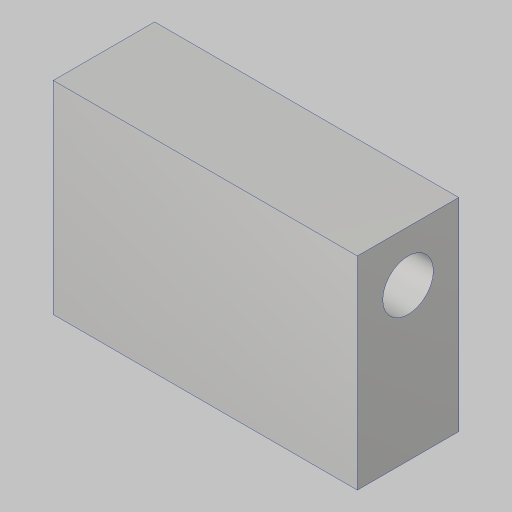
# Autodesk Inventor part: CHD-001
Saved by Autodesk Inventor 2023.5 (Build 275446000, 446)
## iProperties
Created: 2025-01-30
Part Number: CHD-001
Material: Aluminum 6061
Document SubType Name: Modeling
Designer: slick
Density: 2.7 g/cm^3
Appearance: Aluminum - Flat
Author: slick
Autodesk Inventor part; units mm, degrees
ref_plane "YZ Plane" through (0, 0, 0) normal (1, 0, 0) x (0, 1, 0)
ref_plane "XZ Plane" through (0, 0, 0) normal (0, 1, 0) x (-1, 0, 0)
ref_plane "XY Plane" through (0, 0, 0) normal (0, 0, 1) x (1, 0, 0)
sketch "Sketch1" plane through (0, 0, 0) normal (1, 0, 0) x (0, 1, 0)
  line L0 (25.4, 12.7) -> (-25.4, 12.7)
  line L1 (-25.4, 12.7) -> (-25.4, -12.7)
  line L2 (-25.4, -12.7) -> (25.4, -12.7)
  line L3 (25.4, -12.7) -> (25.4, 12.7)
  line L4 (25.4, 12.7) -> (-25.4, -12.7) construction
  line L5 (-25.4, 12.7) -> (25.4, -12.7) construction
  point P0 (0, 0)
  dimension "d0" = 50.8
  dimension "d1" = 25.4
  constraints: 12 end point, 2 midpoint, 2 parallel, 1 horizontal, 1 perpendicular
  measures "d0" distance of L2.end L1.end
  measures "d1" distance of L1.end L0.end
extrude "Extrusion1" add sketch "Sketch1" along normal blind 76.2
sketch "Sketch2" plane through (76.2, 0, 0) normal (1, 0, 0) x (0, 0, -1)
  line L0 (12.7, 25.4) -> (-12.7, 25.4) construction
  point P0 (0, 0)
  point P1 (0, 12.7)
  dimension "d4" = 12.7
  constraints: 1 vertical alignment
  measures "d4" distance from line of L0 point (0, 12.7)
hole "Hole1" at (76.2, 12.7, 0) direction (-1, 0, 0) diameter 12.7 end through all
sketch "Sketch3" plane through (0, -25.4, -12.7) normal (0, -1, 0) x (1, 0, 0)
  line L0 (0, 0) -> (76.2, 0) construction
  line L1 (63.5, 12.7) -> (12.7, 12.7) construction
  line L2 (76.2, 25.4) -> (76.2, 0) construction
  point P0 (0, 12.7)
  point P1 (38.1, 12.7)
  point P2 (38.1, 0)
  point P3 (38.1, 12.7)
  point P4 (76.2, 12.7)
  dimension "d12" = 50.8
  constraints: 3 horizontal alignment, 3 midpoint, 2 end point, 1 coincident, 1 horizontal, 1 vertical alignment
  measures "d12" distance of L1.start L1.end
hole "Hole2" at (63.5, -25.4, 0) at (38.1, -25.4, 0) at (12.7, -25.4, 0) direction (0, 1, 0) diameter 3.9624 depth 25.4 tip angle 118 thread size "10-32 UNF" class "2B" standard "ANSI Unified Screw Threads"
body "Solid1"
